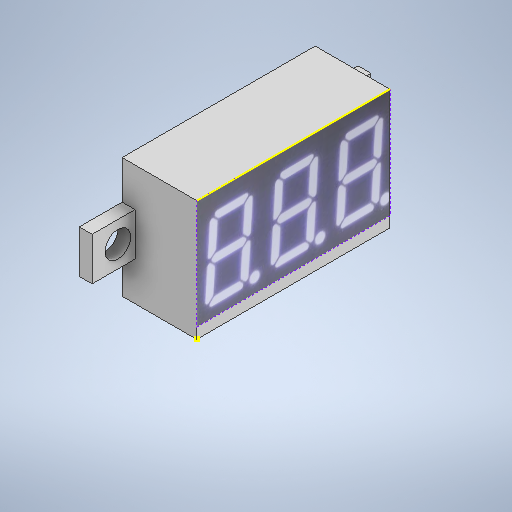
# Autodesk Inventor part: Voltmeter
Saved by Autodesk Inventor 2025.1 (Build 291241000, 241)
## iProperties
Created: 2026-04-17
Part Number: Voltmeter
Material: Generic
Document SubType Name: Modeling
Designer: User
Density: 1 g/cm^3
Appearance: Default
Author: User
Autodesk Inventor part; units mm, degrees
ref_plane "YZ Plane" through (0, 0, 0) normal (1, 0, 0) x (0, 1, 0)
ref_plane "XZ Plane" through (0, 0, 0) normal (0, 1, 0) x (-1, 0, 0)
ref_plane "XY Plane" through (0, 0, 0) normal (0, 0, 1) x (1, 0, 0)
sketch "Sketch1" plane through (0, 0, 0) normal (1, 0, 0) x (0, 1, 0)
  line L0 (0, 0) -> (14, 0)
  line L1 (14, 0) -> (14, -22.5)
  line L2 (14, -22.5) -> (0, -22.5)
  line L3 (0, -22.5) -> (0, 0)
  dimension "d0" = 14
  dimension "d1" = 22.5
  constraints: 8 end point, 2 parallel, 1 horizontal, 1 perpendicular
  measures "d0" distance of L1.end L2.end
  measures "d1" distance of L0.end L1.end
extrude "Extrusion1" add sketch "Sketch1" along normal blind 7.2
sketch "Sketch2" plane through (0, 0, 0) normal (-1, 0, 0) x (0, 0, 1)
  line L0 (-22.5, 0) -> (-22.5, 14) projected
  line L1 (0, 0) -> (-22.5, 0) projected
  line L2 (0, 14) -> (0, 0) projected
  line L3 (-22.5, 14) -> (0, 14) projected
extrude "Extrusion2" add sketch "Sketch2" along normal blind 1.5
sketch "Sketch3" plane through (7.2, 0, 0) normal (0, 0, 1) x (1, 0, 0)
  line L0 (-8.7, 0) -> (-8.7, 14) projected
  line L1 (-8.7, 14) -> (0, 14) projected
  line L2 (-8.7, 0) -> (-7.2, 0)
  line L3 (-7.2, 0) -> (-7.2, 14)
  line L4 (-7.2, 14) -> (-8.7, 14)
  line L5 (-8.7, 14) -> (-8.7, 0)
  line L6 (-8.7, 7) -> (-7.2, 7)
  line L7 (-8.7, 9.5) -> (-7.2, 9.5)
  line L8 (-7.2, 9.5) -> (-7.2, 4.5)
  line L9 (-7.2, 4.5) -> (-8.7, 4.5)
  line L10 (-8.7, 4.5) -> (-8.7, 9.5)
  line L11 (-8.7, 9.5) -> (-7.2, 4.5) construction
  line L12 (-7.2, 9.5) -> (-8.7, 4.5) construction
  point P0 (-7.95, 7)
  dimension "d6" = 5
  constraints: 22 end point, 5 midpoint, 4 parallel, 2 horizontal, 2 perpendicular, 2 point on line
  measures "d6" distance of L7.end L8.end
extrude "Extrusion3" add sketch "Sketch3" along normal blind 5 contours L0 L6 L3 L9 | L0 L7 L3 L6
sketch "Sketch4" plane through (7.2, 0, -22.5) normal (0, 0, -1) x (-1, 0, 0)
  line L0 (8.7, 9.5) -> (8.7, 4.5) projected
  line L1 (8.7, 4.5) -> (7.2, 4.5) projected
  line L2 (7.2, 4.5) -> (7.2, 9.5) projected
  line L3 (7.2, 9.5) -> (8.7, 9.5) projected
  point P0 (7.2, 0)
extrude "Extrusion4" add sketch "Sketch4" along normal blind 5
sketch "Sketch5" plane through (0, 4.5, -22.5) normal (1, 0, 0) x (0, 0, -1)
  line L0 (-22.5, 5) -> (-27.5, 5) projected
  line L1 (-22.5, 0) -> (-27.5, 0) projected
  line L2 (-27.5, 0) -> (-27.5, 5) projected
  line L3 (0, -4.5) -> (0, 9.5) projected
  line L4 (-22.5, 9.5) -> (-22.5, -4.5) projected
  line L5 (0, 5) -> (5, 5) projected
  line L6 (0, 0) -> (5, 0) projected
  line L7 (-27.5, 2.5) -> (-22.5, 2.5)
  line L8 (0, 2.5) -> (5, 2.5)
  line L9 (-22.5, 2.5) -> (-23, 2.5)
  line L10 (0, 2.5) -> (0.5, 2.5)
  line L11 (-23, 2.5) -> (-24.5, 2.5)
  circle A0 centre (-24.5, 2.5) radius 1.5
  line L12 (0.5, 2.5) -> (2, 2.5)
  circle A1 centre (2, 2.5) radius 1.5
  dimension "d11" = 0.5
  dimension "d12" = 0.5
  dimension "d13" = 1.5
  dimension "d14" = 1.5
  constraints: 12 end point, 5 point on line, 3 midpoint, 2 coincident, 2 horizontal alignment, 4 other
  measures "d11" distance of L7.end L9.end
  measures "d12" distance of L8.start L10.end
  measures "d13" distance of L9.end L11.end
  measures "d14" distance of L10.end L12.end
extrude "Extrusion5" cut sketch "Sketch5" against normal blind 5 contours A0 L7 | L7 A0 | A1 L8 | L8 A1
sketch "Sketch6" plane through (7.2, 0, 0) normal (1, 0, 0) x (0, 0, -1)
  line L0 (0, 14) -> (22.5, 14) projected
  line L1 (0, 14) -> (22.6011, 13.9799) construction
  line L2 (22.6011, 13.9799) -> (22.5897, 1.2087) construction
  line L3 (22.5897, 1.2087) -> (-0.0114, 1.2289) construction
  line L4 (-0.0114, 1.2289) -> (0, 14) construction
  point P0 (0, 0)
  constraints: 2 other
body "Solid1"
